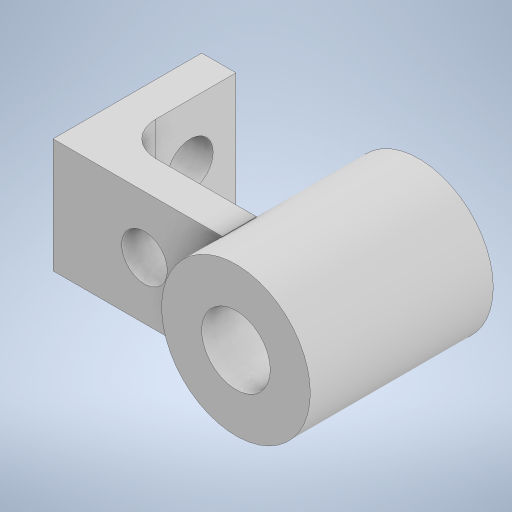
# Autodesk Inventor part: Bartosz_Zukowski_model_nr_10
Saved by Autodesk Inventor 2024 (Build 280153000, 153)
## iProperties
Created: 2024-04-10
Part Number: Bartosz_Zukowski_model_nr_10
Material: Ogólny
Document SubType Name: Modeling
Designer: student156p
Density: 1 g/cm^3
Appearance: Domyślna
Author: student156p
Autodesk Inventor part; units mm, degrees
ref_plane "YZ Plane" through (0, 0, 0) normal (1, 0, 0) x (0, 1, 0)
sketch "Szkic1" plane through (0, 0, 0) normal (0, 0, 1) x (1, 0, 0)
  circle A0 centre (0, 0) radius 15
  circle A1 centre (0, 0) radius 32.5
  dimension "d0" = 65
  dimension "d1" = 30
  constraints: 2 centre point, 2 coincident
  measures "d0" diameter of A1
  measures "d1" diameter of A0
extrude "Wyciągnięcie proste1" add sketch "Szkic1" along normal blind 80
sketch "Szkic2" plane through (0, 0, 0) normal (0, 1, 0) x (-1, 0, 0)
  point P0 (0, 0)
ref_plane "Płaszczyzna konstrukcyjna2" through (0, 32.5, 0) normal (0, 1, 0) x (-1, 0, 0)
sketch "Szkic3" plane through (0, 32.5, 0) normal (0, 1, 0) x (-1, 0, 0)
  line L0 (32.5, 80) -> (-32.5, 80) projected
  line L1 (32.5, 0) -> (-32.5, 0) projected
  line L2 (32.5, 0) -> (32.5, 80) projected
  line L3 (32.5, 0) -> (-32.5, 0) projected
  line L4 (-32.5, 0) -> (-32.5, 80) projected
  line L5 (21, 65) -> (95, 65)
  line L6 (95, 65) -> (95, 0)
  line L7 (95, 0) -> (80, 0)
  line L8 (80, 0) -> (80, 35)
  line L9 (65, 50) -> (21, 50)
  line L10 (21, 50) -> (21, 65)
  arc A0 (80, 35) -> (65, 50) centre (65, 35) ccw
  line L11 (0, 80) -> (0, 0) construction
  dimension "d4" = 15
  dimension "d8" = 15
  dimension "d10" = 65
  dimension "d11" = 65
  dimension "d12" = 95
  dimension "d15" = 15
  constraints: 14 end point, 4 perpendicular, 2 point on circle, 2 tangent, 1 centre point, 1 horizontal, 1 midpoint, 1 parallel, 1 vertical
  measures "d4" radius of A0
  measures "d8" distance between parallel lines of L6 L8
  measures "d10" distance between parallel lines of L5 L1
  measures "d11" distance between parallel lines of L5 L7
  measures "d12" distance between parallel lines of L6 L11
  measures "d15" distance between parallel lines of L9 L5
ref_plane "Płaszczyzna konstrukcyjna3" through (0, 16.25, 0) normal (0, 1, 0) x (-1, 0, 0)
sketch "Szkic4" plane through (0, 0, 0) normal (0, 1, 0) x (-1, 0, 0)
  line L0 (21, 65) -> (95, 65) projected
  line L1 (21, 50) -> (21, 65) projected
  line L2 (65, 50) -> (21, 50) projected
  arc A0 (80, 35) -> (65, 50) centre (65, 35) ccw projected
  line L3 (80, 0) -> (80, 35) projected
  line L4 (95, 65) -> (95, 0) projected
  line L5 (95, 0) -> (80, 0) projected
  point P0 (0, 0)
extrude "Wyciągnięcie proste2" add sketch "Szkic4" along normal mid plane 50
sketch "Szkic5" plane through (-95, -25, 65) normal (-1, 0, 0) x (0, 0, 1)
  circle A0 centre (-45, 25) radius 10
  line L0 (-65, 0) -> (-65, 50) projected
  point P0 (-65, 25)
  dimension "d16" = 20
  dimension "d17" = 20
  constraints: 1 centre point
  measures "d16" diameter of A0
  measures "d17" distance from line of L0 A0.centre
extrude "Wyciągnięcie proste3" cut sketch "Szkic5" against normal blind 50
sketch "Szkic6" plane through (-95, 25, 65) normal (0, 0, 1) x (1, 0, 0)
  circle A0 centre (40, -25) radius 10
  point P0 (95, -25)
  dimension "d20" = 20
  dimension "d21" = 55
  constraints: 1 centre point
  measures "d20" diameter of A0
  measures "d21" distance of point (95, -25) A0.centre
extrude "Wyciągnięcie proste4" cut sketch "Szkic6" against normal blind 50
